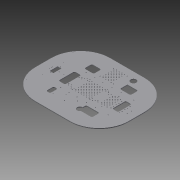
# Autodesk Inventor part: layer 3 update pompa air
Saved by Autodesk Inventor 2013 (Build 170138000, 138)
## iProperties
Created: 2013-01-09
Part Number: layer 3 update pompa air
Material: Generic
Document SubType Name: Modeling
Designer: Irwan Haryanto
Density: 1 g/cm^3
Author: Irwan Haryanto
Autodesk Inventor part; units mm, degrees
ref_plane "YZ Plane" through (0, 0, 0) normal (1, 0, 0) x (0, 1, 0)
ref_plane "XZ Plane" through (0, 0, 0) normal (0, 1, 0) x (-1, 0, 0)
ref_plane "XY Plane" through (0, 0, 0) normal (0, 0, 1) x (1, 0, 0)
sketch "Sketch1" plane through (0, 0, 0) normal (0, 0, 1) x (1, 0, 0)
  circle A0 centre (34.2139, 25.275) radius 1.5
  circle A1 centre (32.9639, 33) radius 1.5
  circle A2 centre (26.2288, 62.5) radius 1.5
  circle A3 centre (75.9639, 32) radius 1.5
  circle A4 centre (26.2288, 113.5) radius 1.5
  circle A5 centre (-34.2861, 25.275) radius 1.5
  arc A6 (-63.0361, 25) -> (-68.0361, 30) centre (-68.0361, 25) ccw
  line L0 (-68.0361, 30) -> (-83.0361, 30)
  arc A7 (-83.0361, 30) -> (-88.0361, 25) centre (-83.0361, 25) ccw
  line L1 (-63.0361, -25) -> (-63.0361, 25)
  circle A8 centre (-34.2861, -25.275) radius 1.5
  arc A9 (-68.0361, -30) -> (-63.0361, -25) centre (-68.0361, -25) ccw
  line L2 (-83.0361, -30) -> (-68.0361, -30)
  arc A10 (-88.0361, -25) -> (-83.0361, -30) centre (-83.0361, -25) ccw
  line L3 (-88.0361, 25) -> (-88.0361, -25)
  line L4 (108.9639, -20.5142) -> (120.9639, -20.5142)
  arc A11 (120.9639, -20.5142) -> (125.9639, -15.5142) centre (120.9639, -15.5142) ccw
  circle A12 centre (34.2139, -25.275) radius 1.5
  arc A13 (103.9639, -15.5142) -> (108.9639, -20.5142) centre (108.9639, -15.5142) ccw
  line L5 (125.9639, -15.5142) -> (125.9639, 25)
  arc A14 (125.9639, 25) -> (120.9639, 30) centre (120.9639, 25) ccw
  line L6 (120.9639, 30) -> (108.9639, 30)
  line L7 (103.9639, 25) -> (103.9639, -15.5142)
  arc A15 (108.9639, 30) -> (103.9639, 25) centre (108.9639, 25) ccw
  circle A16 centre (-33.0361, 33) radius 1.5
  circle A17 centre (-24.7712, 62.5) radius 1.5
  circle A18 centre (-24.7712, 113.5) radius 1.5
  circle A19 centre (-33.0361, -33) radius 1.5
  circle A20 centre (32.9639, -33) radius 1.5
  circle A21 centre (75.9639, -32) radius 1.5
  circle A22 centre (-28.6361, -60.5) radius 1.5
  circle A23 centre (-39.9191, 29.975) radius 1.5
  circle A24 centre (-45.0361, 24.975) radius 1.5
  circle A25 centre (-55.0361, 24.975) radius 1.5
  circle A26 centre (-50.0361, 19.4208) radius 1.5
  circle A27 centre (-60.0361, 19.4208) radius 1.5
  circle A28 centre (-39.9191, -29.975) radius 1.5
  circle A29 centre (-45.0361, -24.975) radius 1.5
  circle A30 centre (-55.0361, -24.975) radius 1.5
  circle A31 centre (-50.0361, -19.4208) radius 1.5
  circle A32 centre (-60.0361, -19.4208) radius 1.5
  circle A33 centre (45.0139, 24.975) radius 1.5
  circle A34 centre (55.0139, 24.975) radius 1.5
  circle A35 centre (39.8968, 29.975) radius 1.5
  circle A36 centre (50.0139, 19.975) radius 1.5
  circle A37 centre (45.0139, -24.975) radius 1.5
  circle A38 centre (55.0139, -24.975) radius 1.5
  circle A39 centre (39.8968, -29.975) radius 1.5
  circle A40 centre (50.0139, -19.975) radius 1.5
  circle A41 centre (-129.0003, 18.1) radius 1.5
  circle A42 centre (-129.0003, -18.1) radius 1.5
  circle A43 centre (-115.0003, 0) radius 1.5
  circle A44 centre (-143.0003, 0) radius 1.5
  line L8 (88.9639, -57.9336) -> (48.9639, -57.9336)
  line L9 (43.9639, -62.9336) -> (43.9639, -70.9336)
  line L10 (53.1969, -86.4336) -> (88.9639, -86.4336)
  line L11 (93.9639, -81.4336) -> (93.9639, -62.9336)
  arc A45 (93.9639, -62.9336) -> (88.9639, -57.9336) centre (88.9639, -62.9336) ccw
  arc A46 (88.9639, -86.4336) -> (93.9639, -81.4336) centre (88.9639, -81.4336) ccw
  arc A47 (48.9639, -57.9336) -> (43.9639, -62.9336) centre (48.9639, -62.9336) ccw
  line L12 (88.9639, 58) -> (58.9639, 58)
  line L13 (53.9639, 63) -> (53.9639, 86.5)
  line L14 (53.9639, 86.5) -> (88.9639, 86.5)
  line L15 (93.9639, 81.5) -> (93.9639, 63)
  arc A48 (93.9639, 81.5) -> (88.9639, 86.5) centre (88.9639, 81.5) ccw
  arc A49 (88.9639, 58) -> (93.9639, 63) centre (88.9639, 63) ccw
  arc A50 (53.9639, 63) -> (58.9639, 58) centre (58.9639, 63) ccw
  line L16 (-73.0361, -57.9336) -> (-68.0361, -57.9336)
  line L17 (-63.0361, -62.9336) -> (-63.0361, -81.4336)
  line L18 (-68.0361, -86.4336) -> (-73.0361, -86.4336)
  line L19 (-78.0361, -81.4336) -> (-78.0361, -62.9336)
  arc A51 (-63.0361, -62.9336) -> (-68.0361, -57.9336) centre (-68.0361, -62.9336) ccw
  arc A52 (-68.0361, -86.4336) -> (-63.0361, -81.4336) centre (-68.0361, -81.4336) ccw
  arc A53 (-78.0361, -81.4336) -> (-73.0361, -86.4336) centre (-73.0361, -81.4336) ccw
  arc A54 (-73.0361, -57.9336) -> (-78.0361, -62.9336) centre (-73.0361, -62.9336) ccw
  line L20 (-74.2712, 58) -> (-49.2712, 58)
  line L21 (-44.2712, 63) -> (-44.2712, 81.5)
  line L22 (-49.2712, 86.5) -> (-74.2712, 86.5)
  line L23 (-79.2712, 81.5) -> (-79.2712, 63)
  arc A55 (-44.2712, 81.5) -> (-49.2712, 86.5) centre (-49.2712, 81.5) ccw
  arc A56 (-49.2712, 58) -> (-44.2712, 63) centre (-49.2712, 63) ccw
  arc A57 (-79.2712, 63) -> (-74.2712, 58) centre (-74.2712, 63) ccw
  arc A58 (-74.2712, 86.5) -> (-79.2712, 81.5) centre (-74.2712, 81.5) ccw
  circle A59 centre (88.9639, 25.5) radius 1.5
  circle A60 centre (88.9639, 5.5) radius 1.5
  circle A61 centre (88.9639, -4.5) radius 1.5
  circle A62 centre (88.9639, -14.5) radius 1.5
  circle A63 centre (88.9639, -24.5) radius 1.5
  circle A64 centre (88.9639, 15.5) radius 1.5
  circle A65 centre (78.9639, 25.5) radius 1.5
  circle A66 centre (83.9639, 20.5) radius 1.5
  circle A67 centre (83.9639, 10.5) radius 1.5
  circle A68 centre (78.9639, 5.5) radius 1.5
  circle A69 centre (83.9639, 0.5) radius 1.5
  circle A70 centre (78.9639, -4.5) radius 1.5
  circle A71 centre (83.9639, -9.5) radius 1.5
  circle A72 centre (78.9639, -14.5) radius 1.5
  circle A73 centre (83.9639, -19.5) radius 1.5
  circle A74 centre (78.9639, -24.5) radius 1.5
  circle A75 centre (78.9639, 15.5) radius 1.5
  circle A76 centre (68.9639, 25.5) radius 1.5
  circle A77 centre (73.9639, 20.5) radius 1.5
  circle A78 centre (73.9639, 10.5) radius 1.5
  circle A79 centre (68.9639, 5.5) radius 1.5
  circle A80 centre (73.9639, 0.5) radius 1.5
  circle A81 centre (68.9639, -4.5) radius 1.5
  circle A82 centre (73.9639, -9.5) radius 1.5
  circle A83 centre (68.9639, -14.5) radius 1.5
  circle A84 centre (73.9639, -19.5) radius 1.5
  circle A85 centre (68.9639, -24.5) radius 1.5
  circle A86 centre (68.9639, 15.5) radius 1.5
  circle A87 centre (63.9639, 20.5) radius 1.5
  circle A88 centre (63.9639, 10.5) radius 1.5
  circle A89 centre (63.9639, 0.5) radius 1.5
  circle A90 centre (63.9639, -9.5) radius 1.5
  circle A91 centre (63.9639, -19.5) radius 1.5
  circle A92 centre (27.9639, 29.5) radius 1.5
  circle A93 centre (27.9639, 9.5) radius 1.5
  circle A94 centre (27.9639, -0.5) radius 1.5
  circle A95 centre (27.9639, -10.5) radius 1.5
  circle A96 centre (27.9639, -20.5) radius 1.5
  circle A97 centre (27.9639, -30.5) radius 1.5
  circle A98 centre (27.9639, 19.5) radius 1.5
  circle A99 centre (17.9639, 29.5) radius 1.5
  circle A100 centre (22.9639, 24.5) radius 1.5
  circle A101 centre (22.9639, 14.5) radius 1.5
  circle A102 centre (17.9639, 9.5) radius 1.5
  circle A103 centre (22.9639, 4.5) radius 1.5
  circle A104 centre (17.9639, -0.5) radius 1.5
  circle A105 centre (22.9639, -5.5) radius 1.5
  circle A106 centre (17.9639, -10.5) radius 1.5
  circle A107 centre (22.9639, -15.5) radius 1.5
  circle A108 centre (17.9639, -20.5) radius 1.5
  circle A109 centre (22.9639, -25.5) radius 1.5
  circle A110 centre (17.9639, -30.5) radius 1.5
  circle A111 centre (17.9639, 19.5) radius 1.5
  circle A112 centre (7.9639, 29.5) radius 1.5
  circle A113 centre (12.9639, 24.5) radius 1.5
  circle A114 centre (12.9639, 14.5) radius 1.5
  circle A115 centre (7.9639, 9.5) radius 1.5
  circle A116 centre (12.9639, 4.5) radius 1.5
  circle A117 centre (7.9639, -0.5) radius 1.5
  circle A118 centre (12.9639, -5.5) radius 1.5
  circle A119 centre (7.9639, -10.5) radius 1.5
  circle A120 centre (12.9639, -15.5) radius 1.5
  circle A121 centre (7.9639, -20.5) radius 1.5
  circle A122 centre (12.9639, -25.5) radius 1.5
  circle A123 centre (7.9639, -30.5) radius 1.5
  circle A124 centre (7.9639, 19.5) radius 1.5
  circle A125 centre (-2.0361, 29.5) radius 1.5
  circle A126 centre (2.9639, 24.5) radius 1.5
  circle A127 centre (2.9639, 14.5) radius 1.5
  circle A128 centre (-2.0361, 9.5) radius 1.5
  circle A129 centre (2.9639, 4.5) radius 1.5
  circle A130 centre (-2.0361, -0.5) radius 1.5
  circle A131 centre (2.9639, -5.5) radius 1.5
  circle A132 centre (-2.0361, -10.5) radius 1.5
  circle A133 centre (2.9639, -15.5) radius 1.5
  circle A134 centre (-2.0361, -20.5) radius 1.5
  circle A135 centre (2.9639, -25.5) radius 1.5
  circle A136 centre (-2.0361, -30.5) radius 1.5
  circle A137 centre (-2.0361, 19.5) radius 1.5
  circle A138 centre (-7.0361, 24.5) radius 1.5
  circle A139 centre (-7.0361, 14.5) radius 1.5
  circle A140 centre (-7.0361, 4.5) radius 1.5
  circle A141 centre (-7.0361, -5.5) radius 1.5
  circle A142 centre (-7.0361, -15.5) radius 1.5
  circle A143 centre (-7.0361, -25.5) radius 1.5
  circle A144 centre (-22.0361, 9.5) radius 1.5
  circle A145 centre (-22.0361, -0.5) radius 1.5
  circle A146 centre (-17.0361, -15.5) radius 1.5
  circle A147 centre (-22.0361, -30.5) radius 1.5
  circle A148 centre (-22.0361, -20.5) radius 1.5
  circle A149 centre (-22.0361, -10.5) radius 1.5
  circle A150 centre (-17.0361, 24.5) radius 1.5
  circle A151 centre (-17.0361, 14.5) radius 1.5
  circle A152 centre (-22.0361, 29.5) radius 1.5
  circle A153 centre (-22.0361, 19.5) radius 1.5
  circle A154 centre (-12.0361, -10.5) radius 1.5
  circle A155 centre (-12.0361, -20.5) radius 1.5
  circle A156 centre (-17.0361, -25.5) radius 1.5
  circle A157 centre (-12.0361, -30.5) radius 1.5
  circle A158 centre (-12.0361, 19.5) radius 1.5
  circle A159 centre (-12.0361, 29.5) radius 1.5
  circle A160 centre (-12.0361, 9.5) radius 1.5
  circle A161 centre (-12.0361, -0.5) radius 1.5
  circle A162 centre (-17.0361, 4.5) radius 1.5
  circle A163 centre (-17.0361, -5.5) radius 1.5
  circle A164 centre (-27.0361, 4.5) radius 1.5
  circle A165 centre (-27.0361, -25.5) radius 1.5
  circle A166 centre (-27.0361, -15.5) radius 1.5
  circle A167 centre (-27.0361, -5.5) radius 1.5
  circle A168 centre (-27.0361, 24.5) radius 1.5
  circle A169 centre (-27.0361, 14.5) radius 1.5
  circle A170 centre (-3.7712, 93.5) radius 1.5
  circle A171 centre (-13.7712, 93.5) radius 1.5
  circle A172 centre (-8.7712, 88.5) radius 1.5
  circle A173 centre (-3.7712, 83.5) radius 1.5
  circle A174 centre (-13.7712, 83.5) radius 1.5
  circle A175 centre (-18.7712, 88.5) radius 1.5
  circle A176 centre (1.2288, 68.5) radius 1.5
  circle A177 centre (-3.7712, 63.5) radius 1.5
  circle A178 centre (-3.7712, 73.5) radius 1.5
  circle A179 centre (-8.7712, 68.5) radius 1.5
  circle A180 centre (-13.7712, 63.5) radius 1.5
  circle A181 centre (-13.7712, 73.5) radius 1.5
  circle A182 centre (-18.7712, 68.5) radius 1.5
  circle A183 centre (-18.7712, 78.5) radius 1.5
  circle A184 centre (1.2288, 108.5) radius 1.5
  circle A185 centre (1.2288, 98.5) radius 1.5
  circle A186 centre (-3.7712, 113.5) radius 1.5
  circle A187 centre (-3.7712, 103.5) radius 1.5
  circle A188 centre (-8.7712, 108.5) radius 1.5
  circle A189 centre (-13.7712, 113.5) radius 1.5
  circle A190 centre (-13.7712, 103.5) radius 1.5
  circle A191 centre (-18.7712, 108.5) radius 1.5
  circle A192 centre (-18.7712, 98.5) radius 1.5
  circle A193 centre (-8.7712, 98.5) radius 1.5
  circle A194 centre (16.2288, 73.5) radius 1.5
  circle A195 centre (16.2288, 63.5) radius 1.5
  circle A196 centre (11.2288, 68.5) radius 1.5
  circle A197 centre (6.2288, 73.5) radius 1.5
  circle A198 centre (6.2288, 63.5) radius 1.5
  circle A199 centre (16.2288, 113.5) radius 1.5
  circle A200 centre (16.2288, 103.5) radius 1.5
  circle A201 centre (11.2288, 108.5) radius 1.5
  circle A202 centre (6.2288, 103.5) radius 1.5
  circle A203 centre (6.2288, 113.5) radius 1.5
  circle A204 centre (16.2288, 93.5) radius 1.5
  circle A205 centre (16.2288, 83.5) radius 1.5
  circle A206 centre (11.2288, 98.5) radius 1.5
  circle A207 centre (6.2288, 93.5) radius 1.5
  circle A208 centre (11.2288, 88.5) radius 1.5
  circle A209 centre (6.2288, 83.5) radius 1.5
  circle A210 centre (11.2288, 78.5) radius 1.5
  circle A211 centre (1.2288, 88.5) radius 1.5
  circle A212 centre (1.2288, 78.5) radius 1.5
  circle A213 centre (-8.7712, 78.5) radius 1.5
  circle A214 centre (68.9639, -47.9336) radius 1.5
  circle A215 centre (68.9639, 48) radius 1.5
  circle A216 centre (116.4639, 48) radius 1.5
  circle A217 centre (116.4639, -47.9336) radius 1.5
  circle A218 centre (-61.7712, 48) radius 1.5
  circle A219 centre (-61.7712, -47.9336) radius 1.5
  circle A220 centre (-98.0361, 0) radius 1.5
  circle A221 centre (-0.2712, -47.9336) radius 1.5
  circle A222 centre (-0.2712, 48) radius 1.5
  circle A223 centre (34.7288, 48) radius 1.5
  circle A224 centre (-30.2712, 48) radius 1.5
  circle A225 centre (34.7288, -47.9336) radius 1.5
  circle A226 centre (-30.2712, -47.9336) radius 1.5
  circle A227 centre (0, 0) radius 0.2438
  arc A228 (43.9639, -70.9336) -> (53.1969, -86.4336) centre (43.9639, -81.4336) ccw
  line L24 (-136.0003, -15) -> (-122.0003, -15)
  line L25 (-122.0003, -15) -> (-122.0003, 15)
  line L26 (-122.0003, 15) -> (-136.0003, 15)
  line L27 (-136.0003, 15) -> (-136.0003, -15)
  circle A229 centre (-145.0003, 6) radius 1
  circle A230 centre (-145.0003, -7) radius 1
  circle A231 centre (147.9639, 8) radius 1.5
  circle A232 centre (147.9639, -8) radius 1.5
  circle A233 centre (-55.0361, -82.5) radius 1.5
  circle A234 centre (13.7639, -60.5) radius 1.5
  circle A235 centre (-12.6361, -82.5) radius 1.5
  circle A236 centre (98.9639, -20) radius 1.5
  circle A237 centre (98.9639, -10) radius 1.5
  circle A238 centre (98.9639, 10) radius 1.5
  circle A239 centre (98.9639, 0) radius 1.5
  circle A240 centre (98.9639, 20) radius 1.5
  circle A241 centre (130.9639, -20) radius 1.5
  circle A242 centre (130.9639, -10) radius 1.5
  circle A243 centre (130.9639, 10) radius 1.5
  circle A244 centre (130.9639, 0) radius 1.5
  circle A245 centre (130.9639, 20) radius 1.5
  line L28 (-175.0003, 0) -> (-0.0005, 0.2438)
  line L29 (-0.0005, 0.2438) -> (-0.0005, 140.2438)
  line L30 (-0.0005, 140.2438) -> (-0.0005, -139.7562)
  line L31 (-0.0005, 140.2438) -> (-65.0005, 140.2438)
  line L32 (-175.0005, 30.2438) -> (-175.0005, -29.7562)
  line L33 (-65.0005, -139.7562) -> (64.9995, -139.7562)
  line L34 (-0.0005, 140.2438) -> (64.9995, 140.2438)
  line L35 (174.9995, 30.2438) -> (174.9995, -29.7562)
  arc A246 (-65.0005, 140.2438) -> (-175.0005, 30.2438) centre (-65.0005, 30.2438) ccw
  arc A247 (174.9995, 30.2438) -> (64.9995, 140.2438) centre (64.9995, 30.2438) ccw
  arc A248 (64.9995, -139.7562) -> (174.9995, -29.7562) centre (64.9995, -29.7562) ccw
  arc A249 (-175.0005, -29.7562) -> (-65.0005, -139.7562) centre (-65.0005, -29.7562) ccw
  line L36 (53.9639, 86.5) -> (53.9639, 81.5)
  line L37 (53.9639, 86.5) -> (58.9639, 86.5)
  arc A250 (58.9639, 86.5) -> (53.9639, 81.5) centre (58.9639, 81.5) ccw
  circle A251 centre (53.9639, 109.2438) radius 10.5
  line L38 (-175.0003, 0) -> (-135.0003, 0)
  line L39 (-175.0003, 0) -> (-135.0003, 0) construction
  line L40 (-88.0361, 30) -> (-65.0003, 30) construction
  circle A252 centre (-137.7567, 39.6126) radius 1
  circle A253 centre (-151.5385, 87.6757) radius 1
  circle A254 centre (-137.6464, -39.5087) radius 1
  circle A255 centre (-151.2943, -87.61) radius 1
  point P0 (0, 0)
  point P1 (103.9639, 30)
  point P2 (-88.0361, 30)
  point P3 (-63.0361, -30)
  point P4 (-88.0361, -30)
  point P5 (125.9639, 30)
  point P6 (43.9639, -86.4336)
  point P7 (93.9639, -86.4336)
  point P8 (53.9639, 58)
  point P9 (93.9639, 86.5)
  point P10 (-44.2712, 86.5)
  point P11 (-79.2712, 86.5)
  point P12 (-175.0005, -139.7562)
  point P13 (174.9995, -139.7562)
  dimension "d51" = 3
  dimension "d54" = 3
  dimension "d64" = 3
  dimension "d69" = 3
  dimension "d76" = 3
  dimension "d77" = 3
  dimension "d78" = 51
  dimension "d82" = 51
  dimension "d90" = 22
  dimension "d91" = 25
  dimension "d92" = 5
  dimension "d94" = 51
  dimension "d96" = 51
  dimension "d116" = 64
  dimension "d117" = 3
  dimension "d118" = 3
  dimension "d119" = 3
  dimension "d120" = 3
  dimension "d121" = 3
  dimension "d122" = 5.633
  dimension "d125" = 4.7
  dimension "d126" = 5
  dimension "d128" = 10
  dimension "d129" = 5
  dimension "d130" = 10
  dimension "d131" = 5
  dimension "d132" = 66
  dimension "d134" = 3
  dimension "d135" = 3
  dimension "d137" = 3
  dimension "d138" = 5.683
  dimension "d139" = 4.7
  dimension "d140" = 5
  dimension "d141" = 10
  dimension "d142" = 5
  dimension "d143" = 3
  dimension "d144" = 5
  dimension "d145" = 5
  dimension "d150" = 3
  dimension "d153" = 3
  dimension "d160" = 36.2
  dimension "d162" = 50
  dimension "d163" = 5
  dimension "d164" = 40
  dimension "d165" = 28.5
  dimension "d166" = 5
  dimension "d170" = 5
  dimension "d171" = 35
  dimension "d172" = 5
  dimension "d177" = 66
  dimension "d182" = 15
  dimension "d184" = 3
  dimension "d185" = 10
  dimension "d186" = 25
  dimension "d187" = 3
  dimension "d188" = 25
  dimension "d189" = 10
  dimension "d190" = 3
  dimension "d196" = 3
  dimension "d197" = 3
  dimension "d198" = 30
  dimension "d199" = 60
  dimension "d200" = 10
  dimension "d201" = 35
  constraints: 255 centre point, 82 end point, 56 point on circle, 54 tangent, 32 point on line, 20 equal radius, 18 parallel, 12 perpendicular, 9 horizontal, 2 symmetric about line, 1 coincident, 1 collinear, 5 other
  measures "d51" diameter of A16
  measures "d54" diameter of A5
  measures "d64" diameter of A22
  measures "d69" diameter of A3
  measures "d76" diameter of A18
  measures "d77" diameter of A17
  measures "d78" distance of A17.centre A18.centre
  measures "d82" distance of A2.centre A4.centre
  measures "d90" distance of point (125.964, 30) point (103.964, 30)
  measures "d91" distance of point (-63.036, -30) point (-88.036, -30)
  measures "d92" radius of A14
  measures "d94" distance of A18.centre A4.centre
  measures "d96" distance of A17.centre A2.centre
  measures "d116" distance of A21.centre A3.centre
  measures "d117" diameter of A23
  measures "d118" diameter of A24
  measures "d119" diameter of A25
  measures "d120" diameter of A26
  measures "d121" diameter of A27
  measures "d122" horizontal distance of A5.centre A23.centre
  measures "d125" vertical distance of A5.centre A23.centre
  measures "d126" vertical distance of A24.centre A23.centre
  measures "d128" distance of A24.centre A25.centre
  measures "d129" vertical distance of A23.centre A25.centre
  measures "d130" distance of A26.centre A27.centre
  measures "d131" horizontal distance of A26.centre A25.centre
  measures "d132" distance of A20.centre A19.centre
  measures "d134" diameter of A33
  measures "d135" diameter of A34
  measures "d137" diameter of A35
  measures "d138" horizontal distance of A35.centre A0.centre
  measures "d139" vertical distance of A35.centre A0.centre
  measures "d140" vertical distance of A33.centre A35.centre
  measures "d141" distance of A34.centre A33.centre
  measures "d142" vertical distance of A34.centre A35.centre
  measures "d143" diameter of A36
  measures "d144" horizontal distance of A36.centre A33.centre
  measures "d145" horizontal distance of A36.centre A33.centre
  measures "d150" diameter of A41
  measures "d153" diameter of A43
  measures "d160" distance of A42.centre A41.centre
  measures "d162" distance of point (93.964, -86.434) point (43.964, -86.434)
  measures "d163" radius of A45
  measures "d164" distance of point (53.964, 86.5) point (93.964, 86.5)
  measures "d165" distance of point (53.964, 58) point (53.964, 86.5)
  measures "d166" radius of A48
  measures "d170" radius of A51
  measures "d171" distance of point (-79.271, 86.5) point (-44.271, 86.5)
  measures "d172" radius of A55
  measures "d177" distance of A20.centre A1.centre
  measures "d182" distance between parallel lines of L19 L17
  measures "d184" diameter of A214
  measures "d185" distance from line of L8 A214.centre
  measures "d186" distance from line of A214.centre L11
  measures "d187" diameter of A215
  measures "d188" distance from line of A215.centre L15
  measures "d189" distance from line of A215.centre L12
  measures "d190" diameter of A216
  measures "d196" diameter of A218
  measures "d197" diameter of A220
  measures "d198" distance from line of A220.centre L0
  measures "d199" distance between parallel lines of L2 L0
  measures "d200" distance from line of A220.centre L3
  measures "d201" distance of A222.centre A223.centre
extrude "Extrusion1" add sketch "Sketch1" along normal blind 3 contours A6 L0 A7 L3 L28 A220 A43 L25 L26 L27 A44 L32 A246 L31 L29 A184 A185 A211 A212 A176 A222 A130 A161 A145 L1 | L28 A145 A161 A130 A227 L30 A221 L33 A249 L32 L38 A44 L27 L24 L25 A43 A220 L3 A10 L2 A9 L1 | L27 L38 A44 L28 | L29 A222 A176 A212 A211 A185 A184 L34 A247 L35 A248 L33 L30 A221 A227 | A44 L38 L28 picked at (-154.6669, 0.0047)
body "Solid1"
